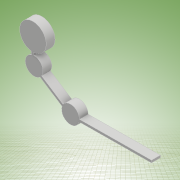
# Autodesk Inventor part: 95thMaleTemplate
Saved by Autodesk Inventor 2017 (Build 210142000, 142)
## iProperties
Created: 2018-03-29
Part Number: 95thMaleTemplate
Material: Generic
Document SubType Name: Modeling
Designer: Spark Electronics
Density: 1 g/cm^3
Appearance: Default
Author: Spark Electronics
Autodesk Inventor part; units mm, degrees
ref_plane "YZ Plane" through (0, 0, 0) normal (1, 0, 0) x (0, 1, 0)
ref_plane "XZ Plane" through (0, 0, 0) normal (0, 1, 0) x (-1, 0, 0)
ref_plane "XY Plane" through (0, 0, 0) normal (0, 0, 1) x (1, 0, 0)
sketch "Sketch1" plane through (0, 0, 0) normal (0, 1, 0) x (-1, 0, 0)
  circle A0 centre (0, 0) radius 150
  circle A1 centre (-13.3087, -279.6835) radius 100
  circle A2 centre (-424.1378, -546.7404) radius 100
  line L0 (0, 0) -> (-13.3087, -279.6835)
  line L1 (-13.3087, -279.6835) -> (-424.1378, -546.7404)
  line L2 (-424.1378, -546.7404) -> (-1339.0994, -538.3521)
  arc A3 (-1324.0769, -381.4083) -> (-1301.514, -806.4251) centre (-424.1378, -546.7404) ccw
  line L3 (25.7594, -1.2258) -> (11.8229, -294.1053)
  line L4 (11.8229, -294.1053) -> (-416.6006, -572.5992)
  line L5 (-416.6006, -572.5992) -> (-1338.9723, -564.1429)
  arc A4 (25.7594, -1.2258) -> (0, 0) centre (12.8797, -0.6129) ccw
  dimension "d0" = 300
  dimension "d1" = 200
  dimension "d2" = 200
  dimension "d3" = 490
  dimension "d4" = 280
  dimension "d10" = 915
  constraints: 12 end point, 6 point on circle, 5 centre point, 2 coincident, 2 tangent, 1 other
  measures "d0" diameter of A0
  measures "d1" diameter of A1
  measures "d2" diameter of A2
  measures "d3" distance of L0.end L1.end
  measures "d4" distance of L0.start L0.end
  measures "d10" radius of A3
extrude "Extrusion1" add sketch "Sketch1" along normal blind 100
body "Solid1"
